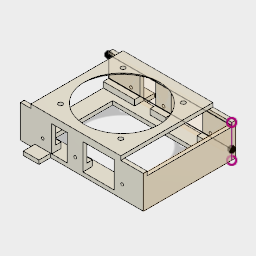
hard-drive-enclosure-v5 (Autodesk Fusion 360 design; units mm, degrees)
Autodesk Fusion 360 part; units mm, degrees
sketch "Sketch1" plane through (0, 0, 0) normal (0, 1, 0) x (1, 0, 0)
  line L0 (68.6494, -55) -> (-78.3404, -55)
  line L1 (-78.3404, -55) -> (-78.3404, 53)
  line L2 (-78.3404, 53) -> (68.6494, 53)
  line L3 (68.6494, 53) -> (68.6494, -55)
  line L4 (78.6494, 58) -> (-78.6124, 58)
  line L5 (-78.6124, 58) -> (-78.6124, -60)
  line L6 (-78.6124, -60) -> (78.6494, -60)
  line L7 (78.6494, -60) -> (78.6494, 58)
  dimension "d1" = 146.9898
  dimension "d2" = 108
  dimension "d3" = 5
  dimension "d4" = 5
  dimension "d5" = 10
  measures "d1" distance of L1 L3
  measures "d2" distance of L0 L2
  measures "d3" distance of L2 L4
  measures "d4" distance of L0 L6
  measures "d5" distance of L3 L7
extrude "Extrude1" add sketch "Sketch1" along normal blind 5 contours L0 L1 L2 L3 | L4 L5 L6 L7
sketch "Sketch2" plane through (0, 5, 0) normal (0, 1, 0) x (-1, 0, 0)
  line L0 (-78.6494, 60) -> (-78.6494, -58)
  line L1 (-78.6494, -58) -> (78.6124, -58)
  line L2 (78.6124, -58) -> (78.6124, 60)
  line L3 (78.6124, 60) -> (-78.6494, 60)
  line L4 (78.6124, -53) -> (-68.6494, -53)
  line L5 (-68.6494, -53) -> (-68.6494, 55)
  line L6 (-68.6494, 55) -> (78.6124, 55)
  line L7 (78.6124, 55) -> (78.6124, -53)
  line L8 (78.6124, -58) -> (-78.6494, -58)
  line L9 (-78.6494, -58) -> (-78.6494, 60)
  line L10 (-78.6494, 60) -> (78.6124, 60)
  line L11 (78.6124, 60) -> (78.6124, -58)
  dimension "d8" = 5
  dimension "d9" = 5
  dimension "d10" = 10
  measures "d8" distance of L1 L4
  measures "d9" distance of L3 L6
  measures "d10" distance of L0 L5
extrude "Extrude2" add sketch "Sketch2" along normal blind 27 contours L0 L1 L2 L3 L4 L5 L6 L8 L9 L10 L11
sketch "Sketch3" plane through (0, 32, 0) normal (0, 1, 0) x (-1, 0, 0)
  line L0 (78.6124, -53) -> (-68.6494, -53)
  line L1 (-68.6494, -53) -> (-68.6494, 55)
  line L2 (-68.6494, 55) -> (78.6124, 55)
  line L3 (78.6124, 55) -> (78.6124, 60)
  line L4 (78.6124, 60) -> (-78.6494, 60)
  line L5 (-78.6494, 60) -> (-78.6494, -58)
  line L6 (-78.6494, -58) -> (78.6124, -58)
  line L7 (78.6124, -58) -> (78.6124, -53)
  line L8 (56.3506, -58) -> (26.3506, -58)
  line L9 (26.3506, -58) -> (26.3506, 60)
  line L10 (26.3506, 60) -> (56.3506, 60)
  line L11 (56.3506, 60) -> (56.3506, -58)
  line L12 (-43.6494, 60) -> (-13.6494, 60)
  line L13 (-13.6494, 60) -> (-13.6494, -58)
  line L14 (-13.6494, -58) -> (-43.6494, -58)
  line L15 (-43.6494, -58) -> (-43.6494, 60)
  dimension "d13" = 112
  dimension "d14" = 30
  dimension "d15" = 30
  dimension "d16" = 40
  dimension "d17" = 25
  measures "d14" distance of L13 L15
  measures "d15" distance of L9 L11
  measures "d16" distance of L9 L13
  measures "d17" distance of L1 L15
extrude "Extrude3" add sketch "Sketch3" along normal blind 10 contours L0 L6 L7 L11 | L0 L6 L8 L9 L11 | L0 L6 L9 L13 | L0 L2 L9 L13 | L2 L3 L4 L11 | L2 L4 L9 L10 L11 | L0 L6 L13 L14 L15 | L2 L4 L9 L13 | L0 L1 L2 L4 L5 L6 L15 | L2 L4 L12 L13 L15
sketch "Sketch4" plane through (0, 0, 0) normal (0, -1, 0) x (1, 0, 0)
  line L0 (78.6494, -58) -> (78.6494, 60)
  line L1 (78.6494, 60) -> (-78.6124, 60)
  line L2 (-78.6124, 60) -> (-78.6124, -58)
  line L3 (-78.6124, -58) -> (78.6494, -58)
  line L4 (-60, 75) -> (-40, 75)
  line L5 (-40, 75) -> (-40, -73)
  line L6 (-40, -73) -> (-60, -73)
  line L7 (-60, -73) -> (-60, 75)
  line L8 (50, -73) -> (30, -73)
  line L9 (30, -73) -> (30, 75)
  line L10 (30, 75) -> (50, 75)
  line L11 (50, 75) -> (50, -73)
  dimension "d20" = 15
  dimension "d21" = 15
  dimension "d22" = 15
  dimension "d23" = 15
  measures "d20" distance of L1 L10
  measures "d21" distance of L3 L8
  measures "d22" distance of L3 L6
  measures "d23" distance of L1 L4
extrude "Extrude4" add sketch "Sketch4" against normal blind 5 contours L3 L8 L9 L11 | L1 L9 L10 L11 | L3 L5 L6 L7 | L1 L4 L5 L7
sketch "Sketch5" plane through (0, 0, 60) normal (0, 0, 1) x (1, 0, 0)
  line L0 (50, 5) -> (50, 0)
  line L1 (50, 0) -> (78.6494, 0)
  line L2 (78.6494, 0) -> (78.6494, 42)
  line L3 (78.6494, 42) -> (-78.6124, 42)
  line L4 (-78.6124, 42) -> (-78.6124, 0)
  line L5 (-78.6124, 0) -> (-60, 0)
  line L6 (-60, 0) -> (-60, 5)
  line L7 (-60, 5) -> (-40, 5)
  line L8 (-40, 5) -> (-40, 0)
  line L9 (-40, 0) -> (30, 0)
  line L10 (30, 0) -> (30, 5)
  line L11 (30, 5) -> (50, 5)
  circle A0 centre (-50.1136, 16.35) radius 1.7525
  circle A1 centre (-8.5084, 16.35) radius 1.7525
  circle A2 centre (51.4864, 16.35) radius 1.7525
  dimension "d26" = 16.35
  dimension "d27" = 16.35
  dimension "d28" = 16.35
  dimension "d29" = 3.505
  dimension "d30" = 3.505
  dimension "d31" = 3.505
  dimension "d32" = 28.4988
  dimension "d33" = 41.6052
  dimension "d34" = 101.6
  measures "d26" distance of L1 A2.centre
  measures "d27" distance of L9 A1.centre
  measures "d28" distance of L9 A0.centre
  measures "d29" diameter of A2
  measures "d30" diameter of A1
  measures "d31" diameter of A0
  measures "d32" distance of L4 A0.centre
  measures "d33" distance of A0.centre A1.centre
  measures "d34" distance of A0.centre A2.centre
extrude "Extrude5" cut sketch "Sketch5" against normal blind 170 contours A0 | A1 | A2
delete_face "DeleteFace1" 1 faces at (43.3333, 5, 65)
delete_face "DeleteFace2" 1 faces at (43.3333, 5, -68)
sketch "Sketch6" plane through (0, 0, 0) normal (0, -1, 0) x (1, 0, 0)
  line L0 (-60, -58) -> (-60, -73)
  line L1 (-60, -73) -> (-40, -73)
  line L2 (-40, -73) -> (-40, -58)
  line L3 (-40, -58) -> (78.6494, -58)
  line L4 (78.6494, -58) -> (78.6494, 60)
  line L5 (78.6494, 60) -> (-40, 60)
  line L6 (-40, 60) -> (-40, 75)
  line L7 (-40, 75) -> (-60, 75)
  line L8 (-60, 75) -> (-60, 60)
  line L9 (-60, 60) -> (-78.6124, 60)
  line L10 (-78.6124, 60) -> (-78.6124, -58)
  line L11 (-78.6124, -58) -> (-60, -58)
  line L12 (-58.6124, 40) -> (58.6494, 40)
  line L13 (58.6494, 40) -> (58.6494, -38)
  line L14 (58.6494, -38) -> (-58.6124, -38)
  line L15 (-58.6124, -38) -> (-58.6124, 40)
  dimension "d37" = 20
  dimension "d38" = 20
  dimension "d39" = 20
  dimension "d40" = 20
  measures "d37" distance of L5 L12
  measures "d38" distance of L3 L14
  measures "d39" distance of L4 L13
  measures "d40" distance of L10 L15
extrude "Extrude6" cut sketch "Sketch6" against normal blind 10 contours L12 L13 L14 L15
sketch "Sketch7" plane through (78.6494, 0, 0) normal (1, 0, 0) x (0, 0, -1)
  line L0 (-60, 0) -> (58, 0)
  line L1 (58, 0) -> (58, 42)
  line L2 (58, 42) -> (-60, 42)
  line L3 (-60, 42) -> (-60, 0)
sketch "Sketch8" plane through (0, 42, 0) normal (0, 1, 0) x (-1, 0, 0)
  line L0 (-13.6494, -53) -> (-68.6494, -53)
  line L1 (-68.6494, -53) -> (-68.6494, 55)
  line L2 (-68.6494, 55) -> (-13.6494, 55)
  line L3 (-13.6494, 55) -> (-13.6494, -53)
  line L4 (-78.6494, -58) -> (78.6124, -58)
  line L5 (78.6124, -58) -> (78.6124, -53)
  line L6 (78.6124, -53) -> (26.3506, -53)
  line L7 (26.3506, -53) -> (26.3506, 55)
  line L8 (26.3506, 55) -> (78.6124, 55)
  line L9 (78.6124, 55) -> (78.6124, 60)
  line L10 (78.6124, 60) -> (-78.6494, 60)
  line L11 (-78.6494, 60) -> (-78.6494, -58)
  line L12 (26.3506, -53) -> (-13.6494, -53)
  line L13 (-13.6494, -53) -> (-13.6494, 55)
  line L14 (-13.6494, 55) -> (26.3506, 55)
  line L15 (26.3506, 55) -> (26.3506, -53)
extrude "Extrude7" cut sketch "Sketch8" against normal blind 15 contours L3 L7 L12 L13 L14 L15
sketch "Sketch9" plane through (0, 0, -53) normal (0, 0, 1) x (1, 0, 0)
  line L0 (68.6494, 42) -> (-78.6124, 42)
  line L1 (-78.6124, 42) -> (-78.6124, 5)
  line L2 (-78.6124, 5) -> (68.6494, 5)
  line L3 (68.6494, 5) -> (68.6494, 42)
  circle A0 centre (-50.1136, 16.35) radius 1.7525
  circle A1 centre (-8.5084, 16.35) radius 1.7525
  circle A2 centre (51.4864, 16.35) radius 1.7525
  line L4 (-78.6124, 38.45) -> (78.6494, 38.45)
  line L5 (78.6494, 38.45) -> (78.6494, 12.35)
  line L6 (78.6494, 12.35) -> (-78.6124, 12.35)
  line L7 (-78.6124, 12.35) -> (-78.6124, 38.45)
  line L8 (78.6494, 0) -> (78.6494, 42)
  dimension "d45" = 26.1
  dimension "d46" = 4
  measures "d45" distance of L4 L6
  measures "d46" distance of A0.centre L6
sketch "Sketch10" plane through (0, 5, 0) normal (0, 1, 0) x (-1, 0, 0)
  line L0 (-58.6494, -38) -> (-58.6494, 40)
  line L1 (-58.6494, 40) -> (58.6124, 40)
  line L2 (58.6124, 40) -> (58.6124, -38)
  line L3 (58.6124, -38) -> (-58.6494, -38)
  line L4 (78.6124, 55) -> (-68.6494, 55)
  line L5 (-68.6494, 55) -> (-68.6494, -53)
  line L6 (-68.6494, -53) -> (78.6124, -53)
  line L7 (78.6124, -53) -> (78.6124, 55)
  line L8 (-68.6494, -53) -> (78.6124, -53)
  line L9 (78.6124, -53) -> (78.6124, -46)
  line L10 (78.6124, -46) -> (-68.6494, -46)
  line L11 (-68.6494, -46) -> (-68.6494, -53)
  line L12 (78.6124, 55) -> (-68.6494, 55)
  line L13 (-68.6494, 55) -> (-68.6494, 48)
  line L14 (-68.6494, 48) -> (78.6124, 48)
  line L15 (78.6124, 48) -> (78.6124, 55)
  dimension "d47" = 7
  dimension "d48" = 7
  measures "d47" distance of L8 L10
  measures "d48" distance of L12 L14
extrude "Extrude8" add sketch "Sketch10" along normal blind 7.25 contours L4 L5 L7 L12 L13 L14 L15 | L5 L6 L7 L8 L9 L10 L11
sketch "Sketch11" plane through (0, 0, 60) normal (0, 0, 1) x (1, 0, 0)
  circle A0 centre (51.4864, 16.35) radius 1.7525
  circle A1 centre (-8.5084, 16.35) radius 1.7525
  circle A2 centre (-50.1136, 16.35) radius 1.7525
  line L0 (78.6494, 42) -> (-78.6124, 42)
  line L1 (-78.6124, 42) -> (-78.6124, 0)
  line L2 (-78.6124, 0) -> (-60, 0)
  line L3 (-60, 0) -> (-60, 5)
  line L4 (-60, 5) -> (-40, 5)
  line L5 (-40, 5) -> (-40, 0)
  line L6 (-40, 0) -> (78.6494, 0)
  line L7 (78.6494, 0) -> (78.6494, 42)
  line L8 (-38.6124, 5) -> (-18.6124, 5)
  line L9 (-18.6124, 5) -> (-18.6124, 38.45)
  line L10 (-18.6124, 38.45) -> (-38.6124, 38.45)
  line L11 (-38.6124, 38.45) -> (-38.6124, 5)
  line L12 (-78.6124, 5) -> (68.6494, 5)
  line L13 (-58.6124, 5) -> (58.6494, 5)
  line L14 (-78.6124, 38.45) -> (78.6494, 38.45)
  line L15 (41.3876, 5) -> (1.3876, 5)
  line L16 (1.3876, 5) -> (1.3876, 38.45)
  line L17 (1.3876, 38.45) -> (41.3876, 38.45)
  line L18 (41.3876, 38.45) -> (41.3876, 5)
  line L19 (-78.6124, 12.35) -> (-78.6124, 38.45)
  dimension "d51" = 20
  dimension "d52" = 40
  dimension "d53" = 20
  dimension "d54" = 40
  measures "d51" distance of L9 L11
  measures "d52" distance of L16 L18
  measures "d53" distance of L9 L16
  measures "d54" distance of L11 L19
extrude "Extrude9" cut sketch "Sketch11" against normal blind 155 contours L12 L13 L14 L15 L16 L17 L18 | L8 L9 L10 L11 L12 L13 L14
sketch "Sketch12" plane through (0, 42, 0) normal (0, 1, 0) x (-1, 0, 0)
  line L0 (78.6124, -53) -> (-68.6494, -53)
  line L1 (-68.6494, -53) -> (-68.6494, 55)
  line L2 (-68.6494, 55) -> (78.6124, 55)
  line L3 (78.6124, 55) -> (78.6124, 60)
  line L4 (78.6124, 60) -> (-78.6494, 60)
  line L5 (-78.6494, 60) -> (-78.6494, -58)
  line L6 (-78.6494, -58) -> (78.6124, -58)
  line L7 (78.6124, -58) -> (78.6124, -53)
  line L8 (55.2661, -46.5) -> (-39.7339, -46.5)
  line L9 (-39.7339, -46.5) -> (-39.7339, 48.5)
  line L10 (-39.7339, 48.5) -> (55.2661, 48.5)
  line L11 (55.2661, 48.5) -> (55.2661, -46.5)
  line L12 (78.6124, -53) -> (-78.6494, -53)
  line L13 (65.2661, -58) -> (-49.7339, -58)
  line L14 (-49.7339, -58) -> (-49.7339, 60)
  line L15 (-49.7339, 60) -> (65.2661, 60)
  line L16 (65.2661, 60) -> (65.2661, -58)
  line L17 (45.2661, -36.5) -> (-29.7339, -36.5)
  line L18 (-29.7339, -36.5) -> (-29.7339, 38.5)
  line L19 (-29.7339, 38.5) -> (45.2661, 38.5)
  line L20 (45.2661, 38.5) -> (45.2661, -36.5)
  circle A0 centre (7.7661, 1) radius 47.5
  point P0 (-49.7339, 60)
  dimension "d57" = 95
  dimension "d58" = 95
  dimension "d59" = 6.5
  dimension "d60" = 3
  dimension "d61" = 10
  dimension "d62" = 10
  dimension "d63" = 18.9155
  dimension "d64" = 10
  dimension "d65" = 10
  dimension "d66" = 10
  dimension "d67" = 10
  dimension "d68" = 87.3958
  measures "d57" distance of L9 L11
  measures "d58" distance of L8 L10
  measures "d59" distance of L2 L10
  measures "d61" distance of L11 L16
  measures "d62" distance of L9 L14
  measures "d63" distance of L1 L14
  measures "d64" distance of L11 L20
  measures "d65" distance of L9 L18
  measures "d66" distance of L8 L17
  measures "d67" distance of L10 L19
extrude "Extrude10" add sketch "Sketch12" along normal blind 5 contours L0 L6 L12 L13 L14 L16 | L0 L2 L12 L14 L16 | L2 L4 L14 L15 L16 | L8 L11 L17 L20 A0 | L8 L9 L17 L18 A0 | L10 L11 L19 L20 A0 | L17 L18 A0 | L17 L20 A0 | L19 L20 A0 | L9 L10 L18 L19 A0 | L18 L19 A0
chamfer "Chamfer1" distance 5 angle 45 1 edges at (36.5194, 42, 18.1767)
chamfer "Chamfer2" distance 10 angle 45 1 edges at (68.6494, 42, 1)
sketch "Sketch13" plane through (0, 42, 0) normal (0, 1, 0) x (-1, 0, 0)
  line L0 (-49.7339, -53) -> (-78.6494, -53)
  line L1 (-78.6494, -53) -> (-78.6494, -58)
  line L2 (-78.6494, -58) -> (-49.7339, -58)
  line L3 (-49.7339, -58) -> (-49.7339, -53)
  line L4 (-78.6494, -53) -> (-68.6494, -53)
  line L5 (-68.6494, -53) -> (-68.6494, 55)
  line L6 (-68.6494, 55) -> (-78.6494, 55)
  line L7 (-78.6494, 55) -> (-78.6494, -53)
  point P0 (-68.6494, 55)
fillet "Fillet1" radius 30 1 edges at (68.6494, 32, 1)
extrude "Extrude11" cut sketch "Sketch13" against normal blind 5 contours L0 L4 L5 L6 L7
sketch "Sketch14" plane through (0, 47, 0) normal (0, 1, 0) x (-1, 0, 0)
  circle A0 centre (7.7661, 1) radius 47.5
  line L0 (65.2661, 60) -> (-49.7339, 60)
  line L1 (-49.7339, 60) -> (-49.7339, -58)
  line L2 (-49.7339, -58) -> (65.2661, -58)
  line L3 (65.2661, -58) -> (65.2661, 60)
  circle A1 centre (46.2661, -39) radius 2.8001
  circle A2 centre (-30.7339, -39) radius 2.8001
  circle A3 centre (-30.7339, 41) radius 2.8001
  circle A4 centre (46.2661, 41) radius 2.8001
  line L4 (55.2661, -46.5) -> (-39.7339, -46.5)
  line L5 (-39.7339, -46.5) -> (-39.7339, 48.5)
  line L6 (-39.7339, 48.5) -> (55.2661, 48.5)
  line L7 (55.2661, 48.5) -> (55.2661, -46.5)
  dimension "d76" = 5.6002
  dimension "d77" = 5.6002
  dimension "d78" = 5.6002
  dimension "d79" = 19
  dimension "d80" = 19
  dimension "d81" = 19
  dimension "d82" = 19
  dimension "d83" = 19
  dimension "d84" = 19
  dimension "d87" = 5.6002
  dimension "d88" = 19
  dimension "d89" = 19
  dimension "d90" = 10
  dimension "d91" = 95
  dimension "d92" = 95
  dimension "d93" = 16.4338
  dimension "d94" = 11.5
  dimension "d95" = 8.07
  dimension "d96" = 4.5
  measures "d76" diameter of A1
  measures "d77" diameter of A2
  measures "d78" diameter of A3
  measures "d79" distance of L0 A3.centre
  measures "d80" distance of L1 A3.centre
  measures "d81" distance of L1 A2.centre
  measures "d82" distance of L2 A2.centre
  measures "d83" distance of L2 A1.centre
  measures "d84" distance of L3 A1.centre
  measures "d87" diameter of A4
  measures "d88" distance of L0 A4.centre
  measures "d89" distance of L3 A4.centre
  measures "d90" distance of L3 L7
  measures "d91" distance of L4.start L6.end
  measures "d92" distance of L5 L7
  measures "d94" distance of L2 L4
extrude "Extrude12" cut sketch "Sketch14" against normal blind 20 contours A1 | A2 | A3 | A4
equation "d4 = d3"
equation "d26 = 0.25 in + 10 mm"
equation "d27 = d26"
equation "d28 = d26"
equation "d30 = d29"
equation "d31 = d29"
equation "d59 = ( 13 / 2 ) * 1 mm"
equation "d65 = d64"
equation "d66 = d64"
equation "d67 = d64"
equation "d77 = d76"
equation "d78 = d76"
equation "d80 = d79"
equation "d81 = d79"
equation "d82 = d79"
equation "d83 = d79"
equation "d84 = d79"
equation "d87 = d76"
equation "d88 = d79"
equation "d89 = d79"
equation "d94 = ( 23 / 2 ) * 1 mm"
